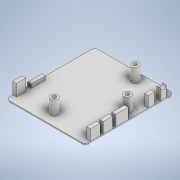
# Autodesk Inventor part: Part1
Saved by Autodesk Inventor 2021 (Build 250183000, 183)
## iProperties
Created: 2021-10-11
Part Number: Part1
Material: Generic
Document SubType Name: Modeling
Designer: Route
Density: 1 g/cm^3
Appearance: Default
Author: Route
Autodesk Inventor part; units mm, degrees
ref_plane "YZ Plane" through (0, 0, 0) normal (1, 0, 0) x (0, 1, 0)
ref_plane "XZ Plane" through (0, 0, 0) normal (0, 1, 0) x (-1, 0, 0)
ref_plane "XY Plane" through (0, 0, 0) normal (0, 0, 1) x (1, 0, 0)
sketch "Sketch1" plane through (0, 0, 0) normal (0, 1, 0) x (-1, 0, 0)
  line L0 (-30, -34) -> (30, -34)
  line L1 (30, -34) -> (30, 34)
  line L2 (30, 34) -> (-30, 34)
  line L3 (-30, 34) -> (-30, -34)
  line L4 (-30, -34) -> (30, 34) construction
  line L5 (30, -34) -> (-30, 34) construction
  line L6 (-33, 37) -> (33, 37)
  line L7 (33, 37) -> (33, -37)
  line L8 (33, -37) -> (-33, -37)
  line L9 (-33, -37) -> (-33, 37)
  line L10 (-33, 37) -> (33, -37) construction
  line L11 (33, 37) -> (-33, -37) construction
  point P0 (0, 0)
  dimension "d0" = 66
  dimension "d1" = 74
  constraints: 24 end point, 4 midpoint, 4 parallel, 2 horizontal, 2 perpendicular
  measures "d0" distance of L7.end L8.end
  measures "d1" distance of L6.end L7.end
extrude "Extrusion1" add sketch "Sketch1" along normal blind 3 contours L3 L2 L1 L0 | L6 L7 L8 L9
sketch "Sketch2" plane through (0, 3, 0) normal (0, 1, 0) x (1, 0, 0)
  line L0 (30, -34) -> (-30, -34)
  line L1 (-30, -34) -> (-30, 34)
  line L2 (-30, 34) -> (30, 34)
  line L3 (30, 34) -> (30, -34)
  line L4 (30, -34) -> (-30, 34) construction
  line L5 (-30, -34) -> (30, 34) construction
  line L6 (33, 37) -> (-33, 37) projected
  line L7 (33, -37) -> (-33, -37)
  line L8 (-33, -37) -> (-33, 37)
  line L9 (-33, 37) -> (33, 37)
  line L10 (33, 37) -> (33, -37)
  line L11 (33, -37) -> (-33, 37) construction
  line L12 (-33, -37) -> (33, 37) construction
  point P0 (0, 0)
  constraints: 24 end point, 4 midpoint, 4 parallel, 2 horizontal, 2 perpendicular
extrude "Extrusion2" add sketch "Sketch2" along normal blind 15
fillet "Fillet1" radius 3 4 edges at (33, 9, 37) (33, 9, -37) (-33, 9, -37) (-33, 9, 37)
fillet "Fillet2" radius 3 8 edges at (-32.1213, 0, 36.1213) (0, 0, 37) (32.1213, 0, 36.1213) (33, 0, 0) (32.1213, 0, -36.1213) (0, 0, -37) (-32.1213, 0, -36.1213) (-33, 0, 0)
sketch "Sketch3" plane through (0, 3, 0) normal (0, 1, 0) x (1, 0, 0)
  arc A0 (33, 34) -> (30, 37) centre (30, 34) ccw projected
  circle A1 centre (8.41, 30.19) radius 1.5
  line L0 (30, 37) -> (30, 34) projected
  circle A2 centre (26.19, 6.06) radius 1.5
  line L1 (-30, -34) -> (30, -34) projected
  circle A3 centre (-3.25, -27.65) radius 1.5
  circle A4 centre (8.41, 30.19) radius 3
  circle A5 centre (-3.25, -27.65) radius 3
  circle A6 centre (26.19, 6.06) radius 3
  point P0 (0, 0)
  dimension "d10" = 3
  dimension "d13" = 3
  dimension "d16" = 3
  dimension "d17" = 6
  dimension "d18" = 6
  dimension "d19" = 6
  constraints: 6 centre point, 3 coincident
  measures "d10" diameter of A1
  measures "d13" diameter of A2
  measures "d16" diameter of A3
  measures "d17" diameter of A4
  measures "d18" diameter of A5
  measures "d19" diameter of A6
extrude "Extrusion3" add sketch "Sketch3" along normal blind 11.4
sketch "Sketch4" plane through (0, 3, 0) normal (0, 1, 0) x (1, 0, 0)
  circle A0 centre (8.41, 30.19) radius 1.5 projected
  circle A1 centre (8.41, 30.19) radius 1.5
  circle A2 centre (26.19, 6.06) radius 1.5 projected
  circle A3 centre (26.19, 6.06) radius 1.5
  circle A4 centre (-3.25, -27.65) radius 1.5 projected
  circle A5 centre (-3.25, -27.65) radius 1.5
  point P0 (0, 0)
  constraints: 3 centre point, 3 coincident
extrude "Extrusion4" cut sketch "Sketch4" against normal blind 3
sketch "Sketch5" plane through (0, 0, 0) normal (0, -1, 0) x (1, 0, 0)
  circle A0 centre (8.41, -30.19) radius 1.5 projected
  circle A1 centre (8.41, -30.19) radius 3
  circle A2 centre (26.19, -6.06) radius 1.5 projected
  circle A3 centre (26.19, -6.06) radius 3
  circle A4 centre (-3.25, 27.65) radius 3 projected
  circle A5 centre (-3.25, 27.65) radius 3
  point P0 (0, 0)
  dimension "d24" = 6
  constraints: 3 centre point, 3 coincident
  measures "d24" diameter of A1
extrude "Extrusion5" cut sketch "Sketch5" against normal blind 2
sketch "Sketch6" plane through (-30, 3, 34) normal (1, 0, 0) x (0, 0, -1)
  line L0 (0, 0) -> (68, 0) projected
  line L1 (0, 0) -> (0, 3.6)
  line L2 (0, 15) -> (0, 0) projected
  line L3 (0, 15) -> (68, 15) projected
  line L4 (68, 0) -> (0, 0) projected
  line L5 (14.44, 3) -> (26.09, 3)
  line L6 (14.44, 3) -> (14.44, 0)
  line L7 (26.09, 3) -> (26.09, 0)
  line L8 (2.54, 4.35) -> (2.54, 0)
  line L9 (10.16, 4.35) -> (10.16, 0)
  line L10 (10.16, 0) -> (10.16, 9.529)
  line L11 (2.54, 0) -> (2.54, 9.529)
  line L12 (2.54, 9.529) -> (10.16, 9.529)
  line L13 (10.16, 0) -> (14.44, 0)
  line L14 (26.09, 0) -> (68, 0)
  line L15 (68, 0) -> (68, 15) projected
  line L16 (68, 0) -> (68, 15)
  line L17 (-3, 15) -> (0, 15) projected
  line L18 (68, 15) -> (0, 15)
  point P0 (34, -3)
  dimension "d27" = 3.6
  dimension "d66" = 9.529
  dimension "d67" = 3
  constraints: 26 end point, 8 perpendicular, 5 point on line, 2 vertical
  measures "d27" distance of L0.start L1.end
  measures "d66" distance of L9.end L10.end
  measures "d67" distance of L5.end L7.end
sketch "Sketch7" plane through (30, 3, -34) normal (-1, 0, 0) x (0, 0, 1)
  line L0 (68, 0) -> (0, 0) projected
  line L1 (68, 0) -> (68, 3.6)
  line L2 (68, 0) -> (68, 15) projected
  line L3 (66.73, 8.861) -> (58.99, 8.861)
  line L4 (48.83, 8.861) -> (56.57, 8.861)
  line L5 (36.25, 8.861) -> (46.41, 8.861)
  line L6 (0, 15) -> (0, 0) projected
  line L7 (0, 0) -> (0, 15) projected
  line L8 (0, 3.6) -> (2.29, 3.6) construction
  arc A0 (5.39, 9.2) -> (9.89, 9.2) centre (7.64, 9.2) ccw
  line L9 (0, 15) -> (68, 15) projected
  line L10 (36.25, 15) -> (46.41, 15)
  line L11 (48.83, 15) -> (56.57, 15)
  line L12 (59, 15) -> (66.73, 15)
  line L13 (9.89, 9.2) -> (9.89, 0)
  line L14 (5.39, 9.2) -> (5.39, 0)
  line L15 (36.25, 8.861) -> (36.25, 0)
  line L16 (46.41, 8.861) -> (46.41, 0)
  line L17 (48.83, 8.861) -> (48.83, 0)
  line L18 (56.57, 8.861) -> (56.57, 0)
  line L19 (58.99, 8.861) -> (58.99, 0)
  line L20 (66.73, 8.861) -> (66.73, 0)
  line L21 (0, 0) -> (68, 0) projected
  line L22 (7.64, 9.2) -> (9.89, 9.2)
  line L23 (9.89, 0) -> (14.761, 0)
  line L24 (14.761, 0) -> (14.761, 8.861)
  line L25 (14.761, 8.861) -> (19.841, 8.861)
  line L26 (19.841, 8.861) -> (19.841, 0)
  point P0 (34, -3)
  point P1 (66.73, 0)
  point P2 (5.39, 0)
  point P3 (9.89, 0)
  point P4 (14.761, 0)
  dimension "d42" = 7.74
  dimension "d43" = 2.42
  dimension "d45" = 2.42
  dimension "d52" = 4.5
  dimension "d70" = 9.2
  dimension "d71" = 8.861
  dimension "d78" = 4.871
  dimension "d79" = 5.08
  dimension "d80" = 90
  constraints: 42 end point, 9 perpendicular, 8 point on line, 3 point on circle, 2 collinear, 2 horizontal, 2 tangent, 1 centre point, 1 parallel, 1 vertical, 4 other
  measures "d42" distance of L3.start L3.end
  measures "d43" distance of L3.end L4.end
  measures "d45" distance of L4.start L5.end
  measures "d52" diameter of A0
  measures "d70" distance of L13.start L13.end
  measures "d71" distance of L5.end L16.end
  measures "d78" distance of L13.end L23.end
  measures "d79" distance of L24.end L25.end
  measures "d80" angle of L24 L25
ref_plane "Work Plane1" through (30, 3, -1) normal (0, 0, -1) x (-1, 0, 0)
split body "Split1" result two bodies by plane through (30, 3, -1) normal (0, 0, -1) first body at (0.1787, 0.5, -11.4817)
move or copy body "Move Body1" bodies to move or copy 2 copy no translate (0, 0, 1.96)
combine bodies "Combine1" operation type add bodies to combine 3 2
ref_plane "Work Plane2" through (3, 3, 34) normal (1, 0, 0) x (0, 0, -1)
split body "Split2" result two bodies by plane through (3, 3, 34) normal (1, 0, 0) bodies 3 first body at (10.9943, 0.5, 1.619)
move or copy body "Move Body2" bodies to move or copy 4 copy no translate (-1.58, 0, 0)
combine bodies "Combine2" operation type add bodies to combine 4 5
extrude "Extrusion8" cut sketch "Sketch6" against normal blind 10 contours L1 L2 L3 L15 L0 L7 L5 L6 L9 L10 L12 L11 L8 bodies 4
extrude "Extrusion9" cut sketch "Sketch7" along normal mid plane 4 contours L0 L20 L3 L19 L18 L4 L17 L16 L5 L15 L26 L25 L24 L13 A0 L14 L6 L9 L2 L1 bodies 4
sketch "Sketch8" plane through (31.42, 3, 34) normal (0, 0, -1) x (-1, 0, 0)
  line L0 (0, 15) -> (3, 15) projected
  arc A0 (61.42, -3) -> (64.42, 0) centre (61.42, 0) ccw projected
  line L1 (0, 15) -> (64.42, 15)
  line L2 (64.42, 15) -> (64.42, 0)
  line L3 (64.42, 0) -> (0, 0)
  line L4 (0, 0) -> (0, 15)
  point P0 (31.42, -3)
  constraints: 8 end point, 2 parallel, 1 horizontal, 1 perpendicular
extrude "Extrusion10" cut sketch "Sketch8" against normal blind 10 bodies 4
sketch "Sketch9" plane through (-30, 3, -32.04) normal (0, 0, 1) x (1, 0, 0)
  line L0 (-2.2712, 0) -> (-2.2712, 15) projected
  line L1 (61.42, 0) -> (58.42, 0) projected
  line L2 (-2.2712, 15) -> (61.42, 15)
  line L3 (61.42, 15) -> (61.42, 0)
  line L4 (61.42, 0) -> (-2.2712, 0)
  line L5 (-2.2712, 0) -> (-2.2712, 15)
  point P0 (30, -3)
  point P1 (58.42, 0)
  constraints: 8 end point, 2 parallel, 1 horizontal, 1 perpendicular
extrude "Extrusion11" cut sketch "Sketch9" against normal blind 10 bodies 4
body "Solid4"
